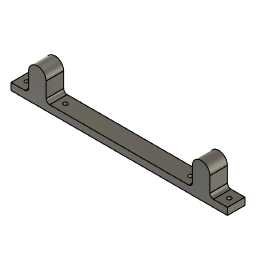
Sestava v22 (Autodesk Fusion 360 archive; units mm, degrees)
design "Držáky vedení X"
Autodesk Fusion 360 part; units mm, degrees
note: some values were not read from the file. Set by a fixed rule: which face or edge a step refers to.
sketch "Bokorys" plane through (0, 0, 0) normal (0, 1, 0) x (1, 0, 0)
  circle A0 centre (0, -22) radius 3
  line L0 (162.5, -6) -> (162.5, 0)
  line L1 (162.5, 0) -> (-22.5, 0)
  line L2 (-22.5, 0) -> (-22.5, -6)
  arc A1 (-7.5, -22) -> (7.5, -22) centre (0, -22) ccw
  line L3 (-22.5, -6) -> (-10.5, -6)
  line L4 (-7.5, -9) -> (-7.5, -22)
  line L5 (7.5, -22) -> (7.5, -9)
  arc A2 (-7.5, -9) -> (-10.5, -6) centre (-10.5, -9) ccw
  arc A3 (10.5, -6) -> (7.5, -9) centre (10.5, -9) ccw
  line L6 (70, 35) -> (70, -50) construction
  arc A4 (132.5, -22) -> (147.5, -22) centre (140, -22) ccw
  circle A5 centre (140, -22) radius 3
  arc A6 (150.5, -6) -> (147.5, -9) centre (150.5, -9) ccw
  line L7 (147.5, -9) -> (147.5, -22)
  line L8 (132.5, -22) -> (132.5, -9)
  arc A7 (132.5, -9) -> (129.5, -6) centre (129.5, -9) ccw
  line L9 (10.5, -6) -> (129.5, -6)
  line L10 (150.5, -6) -> (162.5, -6)
  dimension "d11" = 22
  dimension "d13" = 15
  dimension "d14" = 6
  dimension "d16" = 185
  dimension "d19" = 6
  dimension "d23" = 3
  dimension "d24" = 3
  dimension "d44" = 6
  dimension "d45" = 6
  dimension "d52" = 22.5
  dimension "d53" = 22.5
  dimension "d54" = 92.5
  dimension "d55" = 15
  dimension "d62" = 12.5
  dimension "d72" = 135
  dimension "d73" = 22
  constraint concentric A0 A1
  constraint horizontal L3
  constraint vertical L0
  constraint horizontal L1
  constraint vertical L2
  constraint horizontal L9
  constraint vertical L4
  constraint vertical L5
  constraint tangent L3 A2
  constraint tangent L4 A2
  constraint tangent L5 A3
  constraint tangent A3 L9
  constraint perpendicular L6 L9
  constraint symmetric A0 L6 A5
  constraint symmetric A1 L6 A4
  constraint symmetric A1.start L6 A4.end
  constraint symmetric A1.end L6 A4.start
  constraint symmetric L3.end L6 A6.start
  constraint symmetric L4.start L6 A6.end
  constraint symmetric A2 L6 A6
  constraint symmetric L5.end L6 L8.end
  constraint symmetric A3.start L6 A7.end
  constraint symmetric A3 L6 A7
  constraint collinear L9 L10
  measures "d11" vertical distance of origin A0.centre
  measures "d13" diameter of A1
  measures "d14" diameter of A0
  measures "d16" distance of L0.end L1.end
  measures "d19" vertical distance of origin L2.end
  measures "d23" radius of A2
  measures "d24" radius of A3
  measures "d44" distance of L0.start L0.end
  measures "d45" vertical distance of L2.end L0.end
  measures "d52" horizontal distance of A0.centre L2.end
  measures "d53" distance of origin L1.end
  measures "d54" horizontal distance of L1.end L6.start
  measures "d55" distance of L4 L5
  measures "d73" vertical distance of A0.centre L1.end
extrude "Extrude9" add sketch "Bokorys" along normal blind 15
extrude "Extrude10" add sketch "Bokorys" along normal blind 5 contours A0
extrude "Extrude11" add sketch "Bokorys" along normal blind 5 contours A5
sketch "Sketch6" plane through (0, 0, 0) normal (0, 0, 1) x (1, 0, 0)
  line L0 (-22.5, 0) -> (162.5, 0)
  line L1 (162.5, 0) -> (162.5, 15)
  line L2 (162.5, 15) -> (-22.5, 15)
  line L3 (-22.5, 15) -> (-22.5, 0)
  circle A0 centre (156.5, 7.5) radius 1.75
  line L4 (150.5, 0) -> (162.5, 0)
  circle A1 centre (123.5, 7.5) radius 1.75
  line L5 (70, 42.0713) -> (70, -45) construction
  circle A2 centre (16.5, 7.5) radius 1.75
  circle A3 centre (-16.5, 7.5) radius 1.75
  point P0 (-22.5, 0)
  point P1 (162.5, 15)
  point P2 (162.5, 0)
  point P3 (162.5, 0)
  dimension "d63" = 3.5
  dimension "d64" = 6
  dimension "d65" = 7.5
  dimension "d66" = 3.5
  dimension "d67" = 39
  dimension "d68" = 7.5
  dimension "d69" = 92.5
  constraint horizontal L0
  constraint vertical L1
  constraint horizontal L2
  constraint vertical L3
  constraint coincident P1 L1.end
  constraint coincident P0 L0.start
  constraint vertical L5
  constraint symmetric A0 L5 A3
  constraint symmetric A1 L5 A2
  measures "d63" diameter of A0
  measures "d64" horizontal distance of A0.centre P3
  measures "d65" distance of A0.centre L4
  measures "d66" diameter of A1
  measures "d67" horizontal distance of A1.centre P3
  measures "d68" vertical distance of A1.centre P3
  measures "d69" horizontal distance of P3 L5.end
extrude "Extrude12" cut sketch "Sketch6" along normal blind 15 contours A0 | A1 | A2 | A3
copy_body "Body->Comp1" [suppressed] in component "Component'"
named bodies: "Úchytka"

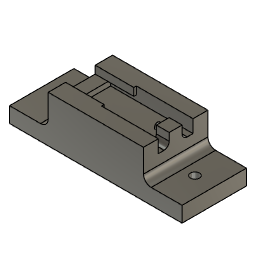
design "Držák napínacího kolečka"
Autodesk Fusion 360 part; units mm, degrees
sketch "Sketch1" plane through (0, 0, 0) normal (1, 0, 0) x (0, 1, 0)
  line L0 (0, 0) -> (25, 0)
  line L1 (25, 0) -> (25, 18)
  line L2 (0, 18) -> (0, 0)
  line L3 (19.25, 15) -> (19.25, 13)
  line L4 (19.25, 13) -> (5.75, 13)
  line L5 (5.75, 13) -> (5.75, 15)
  line L6 (18.25, 18) -> (18.25, 15)
  line L7 (6.75, 15) -> (6.75, 18)
  line L8 (25, 18) -> (18.25, 18)
  line L9 (6.75, 18) -> (0, 18)
  line L10 (5.75, 15) -> (6.75, 15)
  line L11 (18.25, 15) -> (19.25, 15)
  line L12 (6.75, 15) -> (18.25, 15)
  line L13 (5.75, 13) -> (19.25, 13)
  line L14 (19.25, 13) -> (19.25, 18)
  line L15 (19.25, 18) -> (5.75, 18)
  line L16 (5.75, 18) -> (5.75, 13)
  dimension "d1" = 25
  dimension "d2" = 18
  dimension "d3" = 13.5
  dimension "d4" = 2
  dimension "d5" = 13
  dimension "d6" = 5.75
  dimension "d7" = 1
  dimension "d8" = 11.5
  dimension "d9" = 3
  dimension "d10" = 15
  dimension "d32" = 13.5
  constraint horizontal L0
  constraint vertical L1
  constraint horizontal L8
  constraint vertical L2
  constraint coincident L0.start L2.end
  constraint horizontal L10
  constraint vertical L3
  constraint horizontal L4
  constraint vertical L5
  constraint vertical L6
  constraint vertical L7
  constraint collinear L8 L9
  constraint collinear L10 L11
  constraint horizontal L13
  constraint vertical L14
  constraint horizontal L15
  constraint vertical L16
  constraint coincident L8 L14.end
  measures "d1" distance of L0.start L0.end
  measures "d2" distance of L0.end L1.end
  measures "d3" distance of L5.end L3.start
  measures "d4" distance of L3.start L3.end
  measures "d5" vertical distance of L0.start L4.end
  measures "d6" horizontal distance of L0.start L4.end
  measures "d7" horizontal distance of L5.end L7.start
  measures "d8" distance of L6.end L7.start
  measures "d9" distance of L7.end L7.start
  measures "d10" vertical distance of L0.start L7.start
  measures "d32" distance of L14.end L15.end
sketch "Bokorys" plane through (0, 0, 0) normal (0, 1, 0) x (1, 0, 0)
  line L0 (-15, 0) -> (52, 0)
  line L1 (52, 0) -> (52, -6)
  line L2 (-15, -6) -> (-15, 0)
  line L3 (-15, -6) -> (52, -6)
  dimension "d48" = 15
  dimension "d49" = 67
  dimension "d50" = 6
  constraint horizontal L0
  constraint vertical L1
  constraint vertical L2
  constraint horizontal L3
  constraint coincident L2.end L0
  constraint coincident L2 L0.start
  measures "d48" distance of origin L0.start
  measures "d49" distance of L0.end L0.start
  measures "d50" distance of L0.end L1.end
extrude "Extrude1" add sketch "Sketch1" along normal blind 15 contours L0 L1 L2 L3 L4 L5 L8 L9 L13 L14 L16 | L7 L9 L10 L15 L16 | L6 L8 L11 L14 L15 makes body 1
extrude "Extrude2" add sketch "Sketch1" along normal blind 5 contours L3 L4 L5 L10 L11 L12 L13 L14 L16 bodies 1
extrude "Extrude3" add sketch "Sketch1" along normal blind 25 contours L0 L1 L2 L3 L4 L5 L8 L9 L13 L14 L16 bodies 1
extrude "Extrude4" add 1 faces at (25, 10.25, 4.3333) along direction (1, 0, 0) blind 2 on bodies 1 bodies 1
sketch "Sketch4" plane through (27, 0, 0) normal (1, 0, 0) x (0, 1, 0)
  line L0 (0, 18) -> (0, 0)
  line L1 (0, 0) -> (25, 0)
  line L2 (25, 0) -> (25, 18)
  line L3 (25, 18) -> (19.25, 18)
  line L4 (19.25, 18) -> (19.25, 13)
  line L5 (19.25, 13) -> (5.75, 13)
  line L6 (5.75, 13) -> (5.75, 18)
  line L7 (5.75, 18) -> (0, 18)
  line L8 (0, 0) -> (25, 0)
  line L9 (25, 0) -> (25, 18)
  line L10 (25, 18) -> (0, 18)
  line L11 (0, 18) -> (0, 0)
  circle A0 centre (12.5, 15.5) radius 1.25
  line L12 (10, 18) -> (15, 18)
  line L13 (15, 18) -> (15, 13)
  line L14 (15, 13) -> (10, 13)
  line L15 (10, 13) -> (10, 18)
  dimension "d39" = 2.5
  dimension "d40" = 2.5
  dimension "d41" = 25
  dimension "d42" = 12.5
  dimension "d57" = 13
  dimension "d59" = 2.5
  dimension "d60" = 5
  dimension "d61" = 5
  constraint horizontal L8
  constraint vertical L9
  constraint horizontal L10
  constraint vertical L11
  constraint coincident L2.end L3.start
  constraint coincident L0.end L1.start
  constraint horizontal L12
  constraint vertical L13
  constraint horizontal L14
  constraint vertical L15
  measures "d39" diameter of A0
  measures "d40" vertical distance of L4.end A0.centre
  measures "d41" distance of L0.end L1.end
  measures "d42" horizontal distance of A0.centre L0.end
  measures "d57" vertical distance of L0.end L14.end
  measures "d59" horizontal distance of A0.centre L14.end
  measures "d60" distance of L12.start L12.end
  measures "d61" distance of L12.end L13.end
extrude "Extrude5" add sketch "Sketch4" along normal blind 5 separate body contours L0 L1 L2 L3 L4 L5 L6 L7 L8 L9 L10 L11 L14 | L5 L6 L10 L15 | L5 L10 L12 L13 L14 L15 | L4 L5 L10 L13 | A0 makes body 2
extrude "Extrude6" add sketch "Sketch4" against normal blind 3 separate body contours A0 makes body 3
extrude "Extrude7" cut 1 faces at (24, 12.8855, 15.0845) along direction (1, 0, 0) blind 1 on bodies 3 bodies 3
extrude "Extrude8" add sketch "Bokorys" along normal blind 25 separate body makes body 4
combine "Combine1" operation add target body 4 tool bodies 2 1
fillet "Fillet1" radius 3 1 edges at (32, 12.5, 6) on bodies 4
fillet "Fillet2" radius 3 1 edges at (0, 12.5, 6) on bodies 4
extrude "Extrude9" add sketch "Sketch4" along normal blind 5 contours L5 L10 L12 L13 L14 L15 | A0 bodies 3
extrude "Extrude10" cut sketch "Sketch4" along normal blind 5 contours L5 L6 L10 L15 | L4 L5 L10 L13 bodies 4
fillet "Fillet3" radius 2 1 edges at (29.5, 10, 13) on bodies 4
fillet "Fillet4" radius 2 1 edges at (29.5, 15, 13) on bodies 4
combine "Combine2" operation add target body 4 tool bodies 3
move_face "OffsetFaces1" offset 5 1 faces at (32, 1.9167, 13.3333) on bodies 4
move_face "OffsetFaces2" offset -5 1 faces at (27, 12.4689, 17.5822) on bodies 4
move_face "OffsetFaces3" offset -5 1 faces at (25, 12.8855, 15.0845) on bodies 4
sketch "Sketch6" plane through (0, 0, 6) normal (0, 0, 1) x (-1, 0, 0)
  line L0 (3, 0) -> (3, -25)
  line L1 (3, -25) -> (15, -25)
  line L2 (15, -25) -> (15, 0)
  line L3 (15, 0) -> (3, 0)
  line L4 (15, -25) -> (-52, -25)
  line L5 (-52, -25) -> (-52, 0)
  line L6 (-52, 0) -> (15, 0)
  line L7 (15, 0) -> (15, -25)
  circle A0 centre (7.5, -12.5) radius 1.75
  line L8 (-18.5, -37) -> (-18.5, 8) construction
  circle A1 centre (-44.5, -12.5) radius 1.75
  dimension "d73" = 3.5
  dimension "d74" = 12.5
  dimension "d75" = 7.5
  dimension "d76" = 33.5
  dimension "d77" = 67
  constraint horizontal L4
  constraint vertical L5
  constraint horizontal L6
  constraint vertical L7
  constraint coincident L1.end L2.start
  constraint vertical L8
  constraint symmetric A0 L8 A1
  measures "d73" diameter of A0
  measures "d74" vertical distance of origin A0.centre
  measures "d75" horizontal distance of L2.end A0.centre
  measures "d76" distance of L2.end L8
  measures "d77" distance of L1.end L4.end
extrude "Extrude13" cut sketch "Sketch6" against normal blind 16 contours A0 | A1 bodies 4
extrude "Extrude11" [suppressed]
extrude "Extrude12" [suppressed]

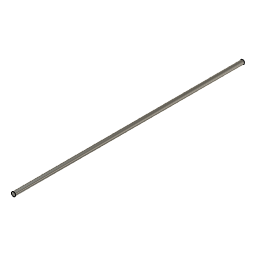
design "Vodící tyč - dlouhá"
Autodesk Fusion 360 part; units mm, degrees
sketch "Sketch1" plane through (0, 0, 0) normal (0, 1, 0) x (1, 0, 0)
  circle A0 centre (0, 0) radius 3
  dimension "d1" = 6
  constraint coincident A0.centre origin
  measures "d1" diameter of A0
extrude "Extrude1" add sketch "Sketch1" along normal blind 336

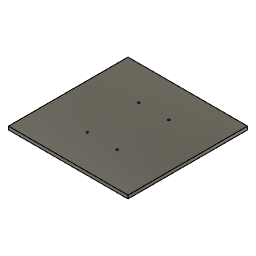
design "Pracovni deska"
Autodesk Fusion 360 part; units mm, degrees
sketch "Sketch1" plane through (0, 0, 0) normal (0, 0, 1) x (1, 0, 0)
  line L0 (0, 0) -> (220, 0)
  line L1 (220, 0) -> (220, 220)
  line L2 (220, 220) -> (0, 220)
  line L3 (0, 220) -> (0, 0)
  circle A0 centre (82.5, 62.5) radius 1.75
  circle A1 centre (137.5, 62.5) radius 1.75
  circle A2 centre (82.5, 157.5) radius 1.75
  circle A3 centre (137.5, 157.5) radius 1.75
  dimension "d3" = 220
  dimension "d5" = 3.5
  dimension "d6" = 82.5
  dimension "d9" = 220
  dimension "d10" = 220
  dimension "d11" = 220
  dimension "d13" = 62.5
  dimension "d16" = 55
  dimension "d17" = 95
  dimension "d18" = 95
  dimension "d19" = 82.5
  constraint horizontal L0
  constraint vertical L1
  constraint horizontal L2
  constraint vertical L3
  measures "d3" distance of L1.end L2.end
  measures "d5" diameter of A0
  measures "d6" horizontal distance of L0.start A0.centre
  measures "d9" distance of L0.start L0.end
  measures "d10" distance of L0.start L2.end
  measures "d11" distance of L0.end L1.end
  measures "d13" vertical distance of L0.start A0.centre
  measures "d19" horizontal distance of L1.end A3.centre
extrude "Extrude1" add sketch "Sketch1" along normal blind 6

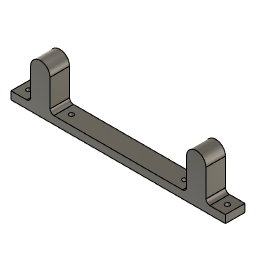
design "Držáky vedení Y"
Autodesk Fusion 360 part; units mm, degrees
sketch "Bokorys" plane through (0, 0, 0) normal (0, 1, 0) x (1, 0, 0)
  circle A0 centre (0, -30) radius 3
  line L0 (142.5, -6) -> (142.5, 0)
  line L1 (142.5, 0) -> (-22.5, 0)
  line L2 (-22.5, 0) -> (-22.5, -6)
  arc A1 (-7.5, -30) -> (7.5, -30) centre (0, -30) ccw
  line L3 (-22.5, -6) -> (-10.5, -6)
  line L4 (-7.5, -9) -> (-7.5, -30)
  line L5 (7.5, -30) -> (7.5, -9)
  arc A2 (-7.5, -9) -> (-10.5, -6) centre (-10.5, -9) ccw
  arc A3 (10.5, -6) -> (7.5, -9) centre (10.5, -9) ccw
  line L6 (60, 35) -> (60, -50) construction
  arc A4 (112.5, -30) -> (127.5, -30) centre (120, -30) ccw
  circle A5 centre (120, -30) radius 3
  arc A6 (130.5, -6) -> (127.5, -9) centre (130.5, -9) ccw
  line L7 (127.5, -9) -> (127.5, -30)
  line L8 (112.5, -30) -> (112.5, -9)
  arc A7 (112.5, -9) -> (109.5, -6) centre (109.5, -9) ccw
  line L9 (10.5, -6) -> (109.5, -6)
  line L10 (130.5, -6) -> (142.5, -6)
  dimension "d11" = 30
  dimension "d13" = 15
  dimension "d14" = 6
  dimension "d16" = 165
  dimension "d19" = 6
  dimension "d23" = 3
  dimension "d24" = 3
  dimension "d44" = 6
  dimension "d45" = 6
  dimension "d52" = 22.5
  dimension "d53" = 22.5
  dimension "d54" = 82.5
  dimension "d55" = 15
  dimension "d62" = 12.5
  dimension "d72" = 135
  constraint concentric A0 A1
  constraint horizontal L3
  constraint vertical L0
  constraint horizontal L1
  constraint vertical L2
  constraint horizontal L9
  constraint vertical L4
  constraint vertical L5
  constraint tangent L3 A2
  constraint tangent L4 A2
  constraint tangent L5 A3
  constraint tangent A3 L9
  constraint perpendicular L6 L9
  constraint symmetric A0 L6 A5
  constraint symmetric A1 L6 A4
  constraint symmetric A1.start L6 A4.end
  constraint symmetric A1.end L6 A4.start
  constraint symmetric L3.end L6 A6.start
  constraint symmetric L4.start L6 A6.end
  constraint symmetric A2 L6 A6
  constraint symmetric L5.end L6 L8.end
  constraint symmetric A3.start L6 A7.end
  constraint symmetric A3 L6 A7
  constraint collinear L9 L10
  measures "d11" vertical distance of origin A0.centre
  measures "d13" diameter of A1
  measures "d14" diameter of A0
  measures "d16" distance of L0.end L1.end
  measures "d19" vertical distance of origin L2.end
  measures "d23" radius of A2
  measures "d24" radius of A3
  measures "d44" distance of L0.start L0.end
  measures "d45" vertical distance of L2.end L0.end
  measures "d52" horizontal distance of A0.centre L2.end
  measures "d53" distance of origin L1.end
  measures "d54" horizontal distance of L1.end L6.start
  measures "d55" distance of L4 L5
extrude "Extrude9" add sketch "Bokorys" along normal blind 15
extrude "Extrude10" add sketch "Bokorys" along normal blind 5 contours A0
extrude "Extrude11" add sketch "Bokorys" along normal blind 5 contours A5
sketch "Sketch6" plane through (0, 0, 0) normal (0, 0, 1) x (1, 0, 0)
  line L0 (-22.5, 0) -> (142.5, 0)
  line L1 (142.5, 0) -> (142.5, 15)
  line L2 (142.5, 15) -> (-22.5, 15)
  line L3 (-22.5, 15) -> (-22.5, 0)
  circle A0 centre (136.5, 7.5) radius 1.75
  line L4 (130.5, 0) -> (142.5, 0)
  circle A1 centre (103.5, 7.5) radius 1.75
  line L5 (60, 42.0713) -> (60, -45) construction
  circle A2 centre (16.5, 7.5) radius 1.75
  circle A3 centre (-16.5, 7.5) radius 1.75
  point P0 (-22.5, 0)
  point P1 (142.5, 15)
  point P2 (142.5, 0)
  point P3 (142.5, 0)
  dimension "d63" = 3.5
  dimension "d64" = 6
  dimension "d65" = 7.5
  dimension "d66" = 3.5
  dimension "d67" = 39
  dimension "d68" = 7.5
  dimension "d69" = 82.5
  dimension "d73" = 165
  dimension "d74" = 153
  dimension "d75" = 87
  constraint horizontal L0
  constraint vertical L1
  constraint horizontal L2
  constraint vertical L3
  constraint coincident P1 L1.end
  constraint coincident P0 L0.start
  constraint vertical L5
  constraint symmetric A0 L5 A3
  constraint symmetric A1 L5 A2
  measures "d63" diameter of A0
  measures "d64" horizontal distance of A0.centre P3
  measures "d65" distance of A0.centre L4
  measures "d66" diameter of A1
  measures "d67" horizontal distance of A1.centre P3
  measures "d68" vertical distance of A1.centre P3
  measures "d69" horizontal distance of P3 L5.end
  measures "d73" distance of P0 P3
  measures "d74" distance of A0.centre A3.centre
  measures "d75" distance of A1.centre A2.centre
extrude "Extrude13" cut sketch "Sketch6" along normal blind 31 contours A0 | A1 | A2 | A3
extrude "Extrude12" [suppressed]
copy_body "Body->Comp1" [suppressed] in component "Úchytka"
equation "d54 = ( 165 / 2 ) * 1 mm"
named bodies: "Úchytka"

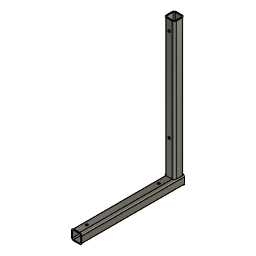
design "Podpěra - jekl"
Autodesk Fusion 360 part; units mm, degrees
sketch "Sketch1" plane through (0, 0, 0) normal (0, 0, 1) x (1, 0, 0)
  line L0 (3, 15) -> (12, 15)
  line L1 (15, 12) -> (15, 3)
  line L2 (12, 0) -> (3, 0)
  line L3 (0, 3) -> (0, 12)
  arc A0 (3, 15) -> (0, 12) centre (3, 12) ccw
  arc A1 (15, 12) -> (12, 15) centre (12, 12) ccw
  arc A2 (12, 0) -> (15, 3) centre (12, 3) ccw
  arc A3 (0, 3) -> (3, 0) centre (3, 3) ccw
  line L4 (3, 13.5) -> (12, 13.5)
  arc A4 (13.5, 12) -> (12, 13.5) centre (12, 12) ccw
  line L5 (13.5, 12) -> (13.5, 3)
  arc A5 (12, 1.5) -> (13.5, 3) centre (12, 3) ccw
  line L6 (12, 1.5) -> (3, 1.5)
  arc A6 (1.5, 3) -> (3, 1.5) centre (3, 3) ccw
  line L7 (1.5, 3) -> (1.5, 12)
  arc A7 (3, 13.5) -> (1.5, 12) centre (3, 12) ccw
  point P0 (0, 15)
  point P1 (15, 15)
  point P2 (15, 0)
  dimension "d1" = 15
  dimension "d2" = 15
  dimension "d3" = 15
  dimension "d4" = 15
  dimension "d5" = 1.5
  dimension "d6" = 3
  constraint horizontal L0
  constraint vertical L1
  constraint horizontal L2
  constraint vertical L3
  constraint coincident P0 L0
  constraint coincident P0 L3
  constraint tangent L0 A0
  constraint tangent L3 A0
  constraint coincident P1 L0
  constraint coincident P1 L1
  constraint tangent L0 A1
  constraint tangent L1 A1
  constraint equal A0 A1
  constraint coincident P2 L1
  constraint coincident P2 L2
  constraint tangent L1 A2
  constraint tangent L2 A2
  constraint equal A0 A2
  constraint coincident origin L2
  constraint coincident origin L3
  constraint tangent L2 A3
  constraint tangent L3 A3
  constraint equal A0 A3
  measures "d1" vertical distance of origin P0
  measures "d2" distance of P0 origin
  measures "d3" distance of origin P2
  measures "d4" distance of P0 P1
  measures "d6" radius of A0
extrude "Extrude1" add sketch "Sketch1" along normal blind 200 makes body 1
sketch "Sketch2" plane through (0, 0, 0) normal (0, 1, 0) x (1, 0, 0)
  line L0 (3, -15) -> (12, -15)
  line L1 (15, -12) -> (15, -3)
  line L2 (12, 0) -> (3, 0)
  line L3 (0, -3) -> (0, -12)
  arc A0 (0, -12) -> (3, -15) centre (3, -12) ccw
  arc A1 (12, -15) -> (15, -12) centre (12, -12) ccw
  arc A2 (15, -3) -> (12, 0) centre (12, -3) ccw
  arc A3 (3, 0) -> (0, -3) centre (3, -3) ccw
  line L4 (3, -13.5) -> (12, -13.5)
  arc A4 (12, -13.5) -> (13.5, -12) centre (12, -12) ccw
  line L5 (13.5, -12) -> (13.5, -3)
  arc A5 (13.5, -3) -> (12, -1.5) centre (12, -3) ccw
  line L6 (12, -1.5) -> (3, -1.5)
  arc A6 (3, -1.5) -> (1.5, -3) centre (3, -3) ccw
  line L7 (1.5, -3) -> (1.5, -12)
  arc A7 (1.5, -12) -> (3, -13.5) centre (3, -12) ccw
  point P0 (0, -15)
  point P1 (15, -15)
  point P2 (15, 0)
  dimension "d9" = 15
  dimension "d10" = 15
  dimension "d11" = 15
  dimension "d12" = 15
  dimension "d13" = -1.5
  dimension "d14" = 3
  constraint horizontal L0
  constraint vertical L1
  constraint horizontal L2
  constraint vertical L3
  constraint coincident P0 L0
  constraint coincident P0 L3
  constraint tangent L0 A0
  constraint tangent L3 A0
  constraint coincident P1 L0
  constraint coincident P1 L1
  constraint tangent L0 A1
  constraint tangent L1 A1
  constraint equal A0 A1
  constraint coincident P2 L1
  constraint coincident P2 L2
  constraint tangent L1 A2
  constraint tangent L2 A2
  constraint equal A0 A2
  constraint tangent L2 A3
  constraint tangent L3 A3
  constraint equal A0 A3
  measures "d9" vertical distance of origin P0
  measures "d10" horizontal distance of origin P2
  measures "d11" distance of P0 P1
  measures "d12" distance of P1 P2
  measures "d14" radius of A0
extrude "Extrude2" add sketch "Sketch2" against normal blind 150 separate body makes body 2
move_body "Move1" bodies 1 to x (1, 0, 0) y (0, 1, 0) z (0, 0, 1) at (0, 0, 15)
move_body "Move2" bodies 2 to x (1, 0, 0) y (0, 1, 0) z (0, 0, 1) at (0, 15, 0)
sketch "Sketch3" plane through (0, 0, 15) normal (0, 0, 1) x (-1, 0, 0)
  line L0 (-12, -15) -> (-3, -15)
  line L1 (-3, -15) -> (-3, 135)
  line L2 (-3, 135) -> (-12, 135)
  line L3 (-12, 135) -> (-12, -15)
  circle A0 centre (-7.5, 15) radius 1.75
  circle A1 centre (-7.5, 120) radius 1.75
  line L4 (-15, -15) -> (-15, 135)
  point P0 (0, 135)
  dimension "d17" = 3.5
  dimension "d18" = 7.5
  dimension "d19" = 15
  dimension "d20" = 5
  dimension "d21" = 3.5
  dimension "d22" = 7.5
  dimension "d23" = 120
  dimension "d24" = 150
  dimension "d25" = 15
  measures "d17" diameter of A0
  measures "d18" horizontal distance of origin A0.centre
  measures "d19" vertical distance of origin A0.centre
  measures "d21" diameter of A1
  measures "d22" horizontal distance of origin A1.centre
  measures "d23" vertical distance of origin A1.centre
  measures "d24" distance of L4.start L4.end
  measures "d25" vertical distance of A1.centre L4.end
extrude "Extrude3" cut sketch "Sketch3" against normal blind 26 contours A0 | A1 bodies 2
sketch "Sketch4" plane through (0, 0, 0) normal (0, -1, 0) x (1, 0, 0)
  line L0 (3, 15) -> (12, 15)
  line L1 (12, 15) -> (12, 215)
  line L2 (12, 215) -> (3, 215)
  line L3 (3, 215) -> (3, 15)
  circle A0 centre (7.5, 200) radius 1.75
  circle A1 centre (7.5, 65) radius 1.75
  dimension "d28" = 3.5
  dimension "d29" = 15
  dimension "d30" = 7.5
  dimension "d31" = 3.5
  dimension "d32" = 7.5
  dimension "d33" = 135
  measures "d28" diameter of A0
  measures "d29" distance of L2 A0.centre
  measures "d30" horizontal distance of origin A0.centre
  measures "d31" diameter of A1
  measures "d32" horizontal distance of origin A1.centre
  measures "d33" distance of A0.centre A1.centre
extrude "Extrude4" cut sketch "Sketch4" against normal blind 35 contours A0 | A1 bodies 1

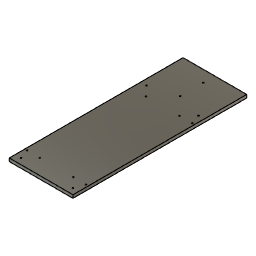
design "Y Deska"
Autodesk Fusion 360 part; units mm, degrees
sketch "Sketch1" plane through (0, 0, 0) normal (0, 0, 1) x (1, 0, 0)
  line L0 (0, 0) -> (165, 0)
  line L1 (165, 0) -> (165, 450)
  line L2 (165, 450) -> (0, 450)
  line L3 (0, 450) -> (0, 0)
  circle A0 centre (6, 40) radius 1.75
  circle A1 centre (159, 40) radius 1.75
  circle A2 centre (159, 40) radius 1.75
  circle A3 centre (159, 315) radius 1.75
  circle A4 centre (39, 40) radius 1.75
  circle A5 centre (126, 40) radius 1.75
  circle A6 centre (39, 315) radius 1.75
  circle A7 centre (126, 315) radius 1.75
  circle A8 centre (15, 15) radius 1.75
  circle A9 centre (6, 315) radius 1.75
  circle A10 centre (159, 315) radius 1.75
  circle A11 centre (150, 15) radius 1.75
  circle A12 centre (15, 340) radius 1.75
  circle A13 centre (150, 340) radius 1.75
  circle A14 centre (82.5, 420) radius 1.75
  circle A15 centre (82.5, 360) radius 1.75
  dimension "d1" = 165
  dimension "d2" = 450
  dimension "d5" = 3.5
  dimension "d6" = 6
  dimension "d7" = 40
  dimension "d10" = 153
  dimension "d11" = 275
  dimension "d14" = 153
  dimension "d15" = 275
  dimension "d17" = 3.5
  dimension "d18" = 40
  dimension "d19" = 39
  dimension "d22" = 0
  dimension "d23" = 0
  dimension "d26" = 87
  dimension "d27" = 275
  dimension "d30" = 3.5
  dimension "d31" = 15
  dimension "d32" = 15
  dimension "d33" = 25
  dimension "d36" = 135
  dimension "d37" = 325
  dimension "d40" = 3.5
  dimension "d41" = 82.5
  dimension "d42" = 420
  dimension "d43" = 3.5
  dimension "d44" = 60
  dimension "d45" = 82.5
  constraint horizontal L0
  constraint vertical L1
  constraint horizontal L2
  constraint vertical L3
  constraint coincident L0.start L3.end
  measures "d1" distance of L0.start L0.end
  measures "d2" distance of L0.start L2.end
  measures "d5" diameter of A0
  measures "d6" horizontal distance of L0.start A0.centre
  measures "d7" vertical distance of L0.start A0.centre
  measures "d17" diameter of A4
  measures "d18" vertical distance of L0.start A4.centre
  measures "d19" horizontal distance of L0.start A4.centre
  measures "d30" diameter of A8
  measures "d31" horizontal distance of L0.start A8.centre
  measures "d32" vertical distance of L0.start A8.centre
  measures "d33" vertical distance of A0.centre A8.centre
  measures "d40" diameter of A14
  measures "d41" horizontal distance of L0.start A14.centre
  measures "d42" vertical distance of L0.start A14.centre
  measures "d43" diameter of A15
  measures "d44" distance of A14.centre A15.centre
  measures "d45" horizontal distance of L2.end A15.centre
extrude "Extrude1" add sketch "Sketch1" along normal blind 8 contours L0 L1 L2 L3 | A0 | A1 A2 | A3 A10 | A4 | A5 | A6 | A7 | A8 | A9 | A11 | A12 | A13 | A14 | A15
extrude "Extrude2" cut sketch "Sketch1" along normal blind 30 contours A0 | A1 A2 | A3 A10 | A4 | A5 | A6 | A7
extrude "Extrude3" cut sketch "Sketch1" along normal blind 25 contours A8 | A11 | A12 | A13
extrude "Extrude4" cut sketch "Sketch1" along normal blind 20 contours A14 | A15

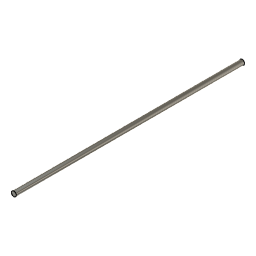
design "Vodící tyč - krátká"
Autodesk Fusion 360 part; units mm, degrees
sketch "Sketch1" plane through (0, 0, 0) normal (0, 1, 0) x (1, 0, 0)
  circle A0 centre (0, 0) radius 3
  dimension "d1" = 6
  constraint coincident A0.centre origin
  measures "d1" diameter of A0
extrude "Extrude1" add sketch "Sketch1" along normal blind 336
extrude "Extrude2" cut 1 faces at (-1.1591, 0, -0.5829) along direction (0, 1, 0) blind 50
extrude "Extrude3" cut 1 faces at (-1.1591, 50, -0.5829) along direction (0, 1, 0) blind 6

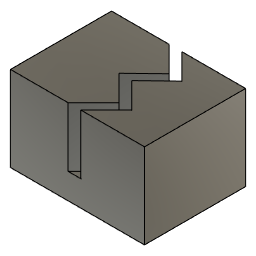
design "Držák řemene"
Autodesk Fusion 360 part; units mm, degrees
sketch "Sketch6" plane through (0, 0, 0) normal (0, 0, 1) x (1, 0, 0)
  line L0 (78, 1.6) -> (70.5, 1.6)
  line L1 (69, 13.5) -> (72, 10.5)
  line L2 (72, 10.5) -> (69, 7.6)
  line L3 (69, 7.6) -> (72, 4.6)
  line L4 (72, 4.6) -> (69, 1.6)
  line L5 (70.5, 13.5) -> (73.5, 10.5)
  line L6 (73.5, 10.5) -> (70.5, 7.6)
  line L7 (73.5, 4.6) -> (70.5, 1.6)
  line L8 (70.5, 7.6) -> (73.5, 4.6)
  line L9 (69, 13.5) -> (62.2186, 13.5)
  line L10 (62.2186, 13.5) -> (62.2186, 1.6)
  line L11 (69, 1.6) -> (62.2186, 1.6)
  line L12 (70.5, 13.5) -> (78, 13.5)
  line L13 (78, 13.5) -> (78, 1.6)
  line L14 (62.2186, 13.5) -> (78, 13.5)
  line L15 (78, 13.5) -> (78, 1.6)
  line L16 (78, 1.6) -> (62.2186, 1.6)
  line L17 (62.2186, 1.6) -> (62.2186, 13.5)
  constraint horizontal L0
  constraint horizontal L9
  constraint vertical L10
  constraint horizontal L11
  constraint vertical L13
  constraint horizontal L12
  constraint coincident L2.start L1
  constraint coincident L2 L1.end
  constraint coincident L3.start L2
  constraint coincident L3 L2.end
  constraint coincident L4.start L3
  constraint coincident L3.end L4
  constraint coincident L5 L6.start
  constraint coincident L5.end L6
  constraint coincident L6 L8.start
  constraint coincident L6.end L8
  constraint coincident L7.start L8
  constraint coincident L8.end L7
  constraint coincident L11 L10.end
  constraint coincident L10 L11.end
  constraint coincident L10 L9.end
  constraint coincident L10.start L9
  constraint coincident L13 L0.start
  constraint coincident L0 L13.end
  constraint horizontal L14
  constraint vertical L15
  constraint horizontal L16
  constraint vertical L17
extrude "Extrude17" add sketch "Sketch6" along normal blind 3 makes body 1
extrude "Extrude18" add sketch "Sketch6" along normal blind 10 separate body contours L0 L5 L6 L7 L8 L12 L13 L14 L15 L16 | L1 L2 L3 L4 L9 L10 L11 L14 L16 L17 makes body 2 at (78, 9.5333, 3.3333) makes body 3 at (62.2186, 5.5667, 6.6667)
combine "Combine1" operation add target body 1 tool bodies 2 3
extrude "Extrude12" [suppressed]
copy_body "Body->Comp1" [suppressed] in component "Úchytka"
named bodies: "Úchytka", "Základna"

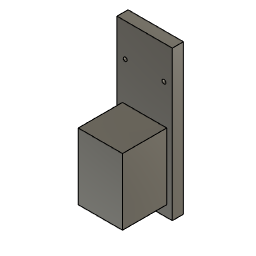
design "Laser Head"
Autodesk Fusion 360 part; units mm, degrees
sketch "Sketch1" plane through (0, 0, 0) normal (0, 0, 1) x (1, 0, 0)
  line L0 (0, 40) -> (40, 40)
  line L1 (40, 40) -> (40, 0)
  line L2 (40, 0) -> (0, 0)
  line L3 (0, 0) -> (0, 40)
  line L4 (-5, 50) -> (45, 50)
  line L5 (45, 50) -> (45, 40)
  line L6 (45, 40) -> (-5, 40)
  line L7 (-5, 40) -> (-5, 50)
  dimension "d1" = 40
  dimension "d2" = 40
  dimension "d3" = 40
  dimension "d4" = 40
  dimension "d5" = 45
  dimension "d6" = 50
  dimension "d7" = 50
  dimension "d8" = 10
  constraint horizontal L0
  constraint vertical L1
  constraint horizontal L2
  constraint vertical L3
  constraint horizontal L4
  constraint vertical L5
  constraint horizontal L6
  constraint vertical L7
  measures "d1" distance of L2.end L0
  measures "d2" distance of L2.end L1
  measures "d3" distance of L0.end L1.end
  measures "d4" distance of L0.start L0.end
  measures "d5" distance of L2.end L5
  measures "d6" distance of L4.start L4.end
  measures "d7" distance of L2.end L4
  measures "d8" distance of L4.start L6.end
extrude "Extrude1" add sketch "Sketch1" along normal blind 60 contours L0 L1 L2 L3 L6 makes body 1
extrude "Extrude2" add sketch "Sketch1" along normal blind 135 separate body contours L0 L4 L5 L6 L7 makes body 2
move_body "Move1" bodies 1 to x (1, 0, 0) y (0, 1, 0) z (0, 0, 1) at (0, 0, 10)
sketch "Sketch2" plane through (0, 50, 0) normal (0, 1, 0) x (-1, 0, 0)
  line L0 (-45, 0) -> (5, 0)
  line L1 (5, 0) -> (5, 135)
  line L2 (5, 135) -> (-45, 135)
  line L3 (-45, 135) -> (-45, 0)
  circle A0 centre (-2.5, 30) radius 1.75
  circle A1 centre (-37.5, 30) radius 1.75
  circle A2 centre (-2.5, 105) radius 1.75
  circle A3 centre (-37.5, 105) radius 1.75
  dimension "d13" = 5
  dimension "d14" = 3.5
  dimension "d15" = 2.5
  dimension "d16" = 30
  dimension "d19" = -35
  dimension "d20" = 75
  measures "d13" distance of origin L0.end
  measures "d14" diameter of A0
  measures "d15" horizontal distance of origin A0.centre
  measures "d16" vertical distance of origin A0.centre
extrude "Extrude3" cut sketch "Sketch2" against normal blind 35 contours A0 | A1 | A2 | A3 bodies 1 2
